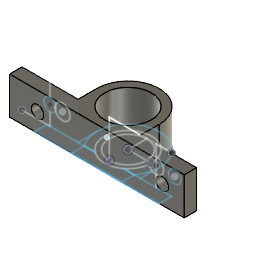
dc motor holder (Autodesk Fusion 360 design; units mm, degrees)
part number: 2026-02-26-00-32-48-952
Autodesk Fusion 360 part; units mm, degrees
note: some values were not read from the file. Set by a fixed rule: which sketch regions a step uses.
sketch "Sketch1" plane through (0, 0, 0) normal (0, 0, 1) x (1, 0, 0)
  circle A0 centre (0, 0) radius 18.75
  line L0 (20, -15) -> (20, -25)
  line L1 (20, -25) -> (-20, -25)
  line L2 (-20, -25) -> (-20, -15)
  line L3 (0, -25) -> (50, -25)
  line L4 (50, -25) -> (-50, -25)
  line L5 (-50, -25) -> (-50, -15)
  line L6 (50, -15) -> (50, -25)
  line L7 (-25, 0) -> (-25, -15)
  line L8 (25, 0) -> (25, -15)
  line L9 (-20, -15) -> (-11.25, -15)
  line L10 (11.25, -15) -> (20, -15)
  arc A1 (20, -15) -> (-20, -15) centre (0, 0) ccw
  line L11 (-20, -15) -> (-11.25, -15)
  line L12 (11.25, -15) -> (20, -15)
  line L13 (-50, -15) -> (-11.25, -15)
  line L14 (11.25, -15) -> (50, -15)
  dimension "d1" = 37.5
  constraint coincident A0.centre A1.centre
  constraint concentric A0 A1
  constraint horizontal L9
  constraint horizontal L11
  constraint vertical L0
  constraint horizontal L1
  constraint vertical L2
  constraint midpoint L1 L3.start
  constraint tangent L3 A1
  constraint perpendicular L0 L3
  constraint horizontal L4
  constraint vertical L5
  constraint horizontal L13
  constraint vertical L6
  constraint coincident L7.start A1
  constraint coincident L7.end L13
  constraint tangent L7 A1
  constraint perpendicular L7 L13
  constraint coincident L8.start A1
  constraint coincident L8.end L14
  constraint tangent L8 A1
  constraint perpendicular L8 L14
  constraint coincident A0 L9.end
  constraint coincident A0 L10.start
  constraint collinear L9 L10
  constraint collinear L11 L12
  constraint collinear L13 L14
  measures "d1" diameter of A0
extrude "Extrude1" add sketch "Sketch1" along normal blind 30 contours A0 L9 L10 A1 L11 L12 L13 L14 | A0 L0 L1 L2 L3 L4 L9 L10 L11 L12 L13 L14 | L7 A1 L13 | L2 L4 L5 L13 | L0 L3 L4 L6 L14 | L8 A1 L14
sketch "Sketch2" plane through (0, 0, 0) normal (0, 0, -1) x (1, 0, 0)
  circle A0 centre (0, 0) radius 18.75
  line L0 (-25, 15) -> (-25, 0)
  arc A1 (-25, 0) -> (25, 0) centre (0, 0) ccw
  line L1 (25, 0) -> (25, 15)
  line L2 (25, 15) -> (50, 15)
  line L3 (50, 15) -> (50, 25)
  line L4 (50, 25) -> (-50, 25)
  line L5 (-50, 25) -> (-50, 15)
  line L6 (-50, 15) -> (-25, 15)
  circle A2 centre (0, 0) radius 15
  line L7 (0, 0) -> (18.75, 0)
  line L8 (18.75, 0) -> (17, 0)
  circle A3 centre (17, 0) radius 1.2
  line L9 (0, 0) -> (0, -15)
  circle A4 centre (-17, 0) radius 1.2
  circle A5 centre (-17, 0) radius 1.5
  circle A6 centre (17, 0) radius 1.5
  dimension "d4" = 30
  dimension "d7" = 2.4
  dimension "d24" = 3
  dimension "d25" = 3
  constraint coincident A0.centre A1.centre
  constraint coincident A0 L7.end
  constraint horizontal L7
  constraint coincident L7 L8.end
  constraint coincident L8.end A3.centre
  constraint coincident A2 L9.end
  constraint perpendicular L7 L9
  constraint symmetric A3 L9 A4
  constraint concentric A4 A5
  constraint concentric A3 A6
  measures "d4" diameter of A2
  measures "d7" diameter of A3
  measures "d24" diameter of A5
  measures "d25" diameter of A6
extrude "Extrude3" add sketch "Sketch2" against normal blind 2.4 contours A0 | L7 L8 A3 A6 | L7 L8 A3 A6 | A5
sketch "Sketch3" plane through (0, -15, 0) normal (0, 1, 0) x (-1, 0, 0)
  line L0 (-50, 0) -> (-25, 0)
  line L1 (-25, 0) -> (-25, 30)
  line L2 (-25, 30) -> (-50, 30)
  line L3 (-50, 30) -> (-50, 0)
  line L4 (-50, 30) -> (-37.5, 30)
  line L5 (-37.5, 0) -> (-37.5, 30)
  circle A0 centre (-37.5, 15) radius 6
  line L6 (-50, 30) -> (0, 30)
  line L7 (0, 30) -> (0, 0)
  circle A1 centre (37.5, 15) radius 6
  dimension "d10" = 12
  constraint coincident L2.end L3.start
  constraint midpoint L2 L4.end
  constraint midpoint L0 L5.start
  constraint midpoint L5 A0.centre
  constraint perpendicular L3 L6
  constraint coincident L7.end origin
  constraint perpendicular L6 L7
  constraint symmetric A0 L7 A1
  measures "d10" diameter of A0
extrude "Extrude5" add 1 faces at (50, -18.3333, 10) along direction (1, 0, 0) blind 20
extrude "Extrude6" add 1 faces at (-50, -21.6667, 10) along direction (-1, 0, 0) blind 20
sketch "Sketch4" plane through (0, -15, 0) normal (0, 1, 0) x (-1, 0, 0)
  line L0 (25, 0) -> (70, 0)
  line L1 (70, 0) -> (70, 30)
  line L2 (70, 30) -> (25, 30)
  line L3 (25, 30) -> (25, 0)
  line L4 (70, 0) -> (47.5, 0)
  circle A0 centre (47.5, 15) radius 5
  circle A1 centre (-52.5, 15) radius 5
  line L5 (47.5, 0) -> (47.5, 10)
  line L6 (47.5, 20) -> (47.5, 30)
  dimension "d19" = 10
  dimension "d20" = 100
  dimension "d21" = 10
  constraint coincident L0.end L1.start
  constraint midpoint L0 L4.end
  constraint midpoint L2 L6.end
  constraint coincident A0 L5.end
  constraint coincident A0 L6.start
  constraint collinear L5 L6
  constraint coincident A0.centre L5
  measures "d19" diameter of A0
  measures "d20" distance of A0.centre A1.centre
  measures "d21" diameter of A1
extrude "Extrude7" cut sketch "Sketch4" against normal blind 24 contours A0 | A1
extrude "Extrude8" cut sketch "Sketch2" against normal blind 26 contours A5
extrude "Extrude9" cut sketch "Sketch2" against normal blind 40 contours L7 L8 A3 A6 | L7 L8 A3 A6
